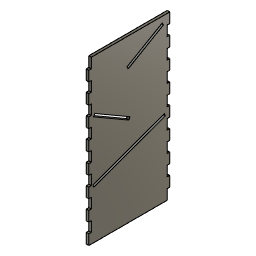
Dice Tower (Right Side) (Autodesk Fusion 360 design; units mm, degrees)
Autodesk Fusion 360 part; units mm, degrees
note: some values were not read from the file. Set by a fixed rule: which sketch regions a step uses.
sketch "Sketch1" plane through (0, 0, 0) normal (1, 0, 0) x (0, 1, 0)
  line L0 (98.425, 139.7) -> (101.6, 139.7)
  line L1 (0, 101.6) -> (0, 114.3)
  line L2 (0, 127) -> (0, 139.7)
  line L3 (98.425, 114.3) -> (101.6, 114.3)
  line L4 (0, 127) -> (3.175, 127)
  line L5 (101.6, 101.6) -> (101.6, 88.9)
  line L6 (0, 101.6) -> (3.175, 101.6)
  line L7 (98.425, 0) -> (98.425, 203.2)
  line L8 (98.425, 114.3) -> (98.425, 101.6)
  line L9 (98.425, 88.9) -> (101.6, 88.9)
  line L10 (101.6, 0) -> (100.0125, 0)
  line L11 (98.425, 127) -> (101.6, 127)
  line L12 (98.425, 101.6) -> (101.6, 101.6)
  line L13 (98.425, 95.25) -> (98.425, 88.9)
  line L14 (3.175, 0) -> (3.175, 203.2)
  line L15 (101.6, 127) -> (101.6, 114.3)
  line L16 (3.175, 127) -> (3.175, 114.3)
  line L17 (3.175, 88.9) -> (0, 88.9)
  line L18 (98.425, 139.7) -> (98.425, 127)
  line L19 (3.175, 114.3) -> (0, 114.3)
  line L20 (3.175, 12.7) -> (3.175, 0)
  line L21 (3.175, 190.5) -> (3.175, 177.8)
  line L22 (3.175, 177.8) -> (0, 177.8)
  line L23 (101.6, 50.8) -> (101.6, 38.1)
  line L24 (3.175, 50.8) -> (3.175, 38.1)
  line L25 (98.425, 152.4) -> (101.6, 152.4)
  line L26 (98.425, 50.8) -> (101.6, 50.8)
  line L27 (98.425, 152.4) -> (98.425, 139.7)
  line L28 (3.175, 139.7) -> (0, 139.7)
  line L29 (0, 139.7) -> (0, 127)
  line L30 (3.175, 101.6) -> (3.175, 88.9)
  line L31 (98.425, 101.6) -> (98.425, 95.25)
  line L32 (98.425, 203.2) -> (98.425, 190.5)
  line L33 (101.6, 152.4) -> (101.6, 139.7)
  line L34 (101.6, 203.2) -> (101.6, 190.5)
  line L35 (3.175, 203.2) -> (3.175, 190.5)
  line L36 (0, 0) -> (11.0998, 0)
  line L37 (98.425, 177.8) -> (98.425, 165.1)
  line L38 (98.425, 127) -> (98.425, 114.3)
  line L39 (0, 165.1) -> (0, 152.4)
  line L40 (11.0998, 0) -> (6.0198, 0)
  line L41 (98.425, 88.9) -> (98.425, 76.2)
  line L42 (0, 38.1) -> (3.175, 38.1)
  line L43 (98.425, 38.1) -> (98.425, 25.4)
  line L44 (101.6, 177.8) -> (101.6, 165.1)
  line L45 (98.425, 12.7) -> (101.6, 12.7)
  line L46 (0, 177.8) -> (0, 190.5)
  line L47 (98.425, 177.8) -> (101.6, 177.8)
  line L48 (0, 76.2) -> (0, 88.9)
  line L49 (0, 114.3) -> (0, 101.6)
  line L50 (3.175, 190.5) -> (0, 190.5)
  line L51 (98.425, 190.5) -> (101.6, 190.5)
  line L52 (101.6, 0) -> (0, 0)
  line L53 (98.425, 38.1) -> (101.6, 38.1)
  line L54 (90.5002, 0) -> (95.5802, 0)
  line L55 (3.175, 203.2) -> (101.6, 203.2)
  line L56 (98.425, 76.2) -> (101.6, 76.2)
  line L57 (98.425, 165.1) -> (101.6, 165.1)
  line L58 (98.425, 63.5) -> (98.425, 50.8)
  line L59 (98.425, 25.4) -> (101.6, 25.4)
  line L60 (0, 0) -> (0, 12.7)
  line L61 (3.175, 63.5) -> (0, 63.5)
  line L62 (98.425, 63.5) -> (101.6, 63.5)
  line L63 (0, 152.4) -> (0, 165.1)
  line L64 (0, 152.4) -> (3.175, 152.4)
  line L65 (0, 25.4) -> (0, 38.1)
  line L66 (0, 0) -> (12.065, 0)
  line L67 (3.175, 50.8) -> (0, 50.8)
  line L68 (101.6, 203.2) -> (98.425, 203.2)
  line L69 (98.425, 190.5) -> (98.425, 177.8)
  line L70 (101.6, 76.2) -> (101.6, 63.5)
  line L71 (101.6, 0) -> (90.5002, 0)
  line L72 (3.175, 25.4) -> (3.175, 12.7)
  line L73 (98.425, 25.4) -> (98.425, 12.7)
  line L74 (3.175, 38.1) -> (3.175, 25.4)
  line L75 (0, 12.7) -> (3.175, 12.7)
  line L76 (0, 50.8) -> (0, 63.5)
  line L77 (0, 25.4) -> (3.175, 25.4)
  line L78 (3.175, 177.8) -> (3.175, 165.1)
  line L79 (101.6, 0) -> (98.425, 0)
  line L80 (101.6, 0) -> (85.725, 0)
  line L81 (101.6, 25.4) -> (101.6, 12.7)
  line L82 (3.175, 76.2) -> (0, 76.2)
  line L83 (98.425, 165.1) -> (98.425, 152.4)
  line L84 (3.175, 63.5) -> (3.175, 50.8)
  line L85 (3.175, 152.4) -> (3.175, 139.7)
  line L86 (98.425, 76.2) -> (98.425, 63.5)
  line L87 (3.175, 165.1) -> (0, 165.1)
  line L88 (98.425, 50.8) -> (98.425, 38.1)
  line L89 (3.175, 76.2) -> (3.175, 63.5)
  line L90 (0, 0) -> (3.175, 0)
  line L91 (3.175, 88.9) -> (3.175, 76.2)
  line L92 (98.425, 203.2) -> (98.425, 177.8)
  line L93 (3.175, 0) -> (3.175, 59.055)
  line L94 (7.62, 139.7) -> (51.5837, 114.2474)
  line L95 (49.9801, 111.4777) -> (6.0165, 136.9303)
  line L96 (6.0165, 136.9303) -> (7.62, 139.7)
  line L97 (93.7411, 193.04) -> (49.7434, 167.6463)
  line L98 (92.1413, 195.8119) -> (93.7411, 193.04)
  line L99 (48.1436, 170.4182) -> (92.1413, 195.8119)
  line L100 (3.175, 60.2676) -> (4.1957, 60.2676)
  line L101 (4.1957, 60.2676) -> (6.35, 60.2676)
  line L102 (6.35, 60.2676) -> (95.8689, 92.8088)
  line L103 (94.7755, 95.8167) -> (5.2566, 63.2754)
  line L104 (49.9801, 111.4777) -> (50.2, 111.3504)
  line L105 (50.2, 111.3504) -> (51.8035, 114.1201)
  line L106 (51.8035, 114.1201) -> (51.5837, 114.2474)
  line L107 (95.8689, 92.8088) -> (96.1076, 92.8956)
  line L108 (96.1076, 92.8956) -> (95.0142, 95.9034)
  line L109 (95.0142, 95.9034) -> (94.7755, 95.8167)
  line L110 (49.7434, 167.6463) -> (49.5234, 167.5194)
  line L111 (49.5234, 167.5194) -> (47.9236, 170.2912)
  line L112 (47.9236, 170.2912) -> (48.1436, 170.4182)
  line L113 (5.2566, 63.2754) -> (6.35, 60.2676)
  dimension "d9" = 11.0998
  dimension "d10" = 11.0998
  dimension "d14" = 5.08
  dimension "d15" = 5.08
  dimension "d27" = 3.175
  dimension "d28" = 3.175
  dimension "d40" = 3.175
  dimension "d41" = 3.175
  dimension "d42" = 12.7
  dimension "d43" = 12.7
  dimension "d44" = 12.7
  dimension "d45" = 12.7
  dimension "d46" = 12.7
  dimension "d47" = 12.7
  dimension "d48" = 12.7
  dimension "d49" = 12.7
  dimension "d50" = 6.35
  dimension "d51" = 6.35
  dimension "d52" = 12.7
  dimension "d53" = 12.7
  dimension "d54" = 12.7
  dimension "d55" = 12.7
  dimension "d56" = 12.7
  dimension "d57" = 12.7
  dimension "d74" = 59.055
  dimension "d78" = 50.8
  dimension "d79" = 3.2004
  dimension "d80" = 50.8
  dimension "d81" = 50.8
  dimension "d82" = 3.2004
  dimension "d83" = 50.8
  dimension "d84" = 95.25
  dimension "d85" = 3.2004
  dimension "d86" = 95.25
  dimension "d87" = 0.254
  dimension "d88" = 0.254
  dimension "d89" = 3.2004
  dimension "d90" = 0.254
  dimension "d91" = 3.2004
  constraint coincident L36.start L52.end
  constraint vertical L60
  constraint perpendicular L55 L60
  constraint perpendicular L34 L55
  constraint perpendicular L52 L60
  constraint perpendicular L60 L66
  constraint perpendicular L34 L80
  constraint perpendicular L10 L34
  constraint coincident L54.start L52
  constraint perpendicular L36 L60
  constraint perpendicular L50 L60
  constraint perpendicular L21 L50
  constraint coincident L22.end L60
  constraint perpendicular L22 L60
  constraint perpendicular L22 L78
  constraint perpendicular L60 L87
  constraint collinear L46 L60
  constraint perpendicular L39 L87
  constraint perpendicular L39 L64
  constraint parallel L66 L90
  constraint perpendicular L14 L55
  constraint perpendicular L64 L85
  constraint perpendicular L28 L60
  constraint perpendicular L28 L29
  constraint coincident L4.end L14
  constraint perpendicular L4 L14
  constraint perpendicular L4 L16
  constraint perpendicular L16 L19
  constraint perpendicular L19 L49
  constraint midpoint L6.end L14
  constraint perpendicular L6 L14
  constraint perpendicular L6 L30
  constraint parallel L14 L91
  constraint parallel L14 L89
  constraint parallel L14 L84
  constraint parallel L14 L24
  constraint parallel L24 L74
  constraint parallel L14 L72
  constraint perpendicular L17 L60
  constraint coincident L48.start L60
  constraint perpendicular L60 L82
  constraint perpendicular L60 L61
  constraint coincident L67.end L60
  constraint perpendicular L60 L67
  constraint coincident L65.start L60
  constraint collinear L60 L63
  constraint collinear L2 L60
  constraint collinear L1 L60
  constraint collinear L48 L60
  constraint collinear L60 L76
  constraint collinear L60 L65
  constraint perpendicular L34 L68
  constraint perpendicular L34 L79
  constraint perpendicular L32 L55
  constraint perpendicular L34 L51
  constraint perpendicular L51 L69
  constraint coincident L44.start L34
  constraint perpendicular L34 L47
  constraint perpendicular L37 L47
  constraint coincident L44.end L34
  constraint perpendicular L34 L57
  constraint perpendicular L57 L83
  constraint coincident L25.end L34
  constraint perpendicular L25 L34
  constraint perpendicular L25 L27
  constraint coincident L0.end L34
  constraint perpendicular L0 L34
  constraint perpendicular L0 L18
  constraint coincident L11.end L34
  constraint perpendicular L11 L34
  constraint perpendicular L11 L38
  constraint coincident L3.end L34
  constraint perpendicular L3 L34
  constraint perpendicular L3 L8
  constraint perpendicular L12 L34
  constraint perpendicular L12 L31
  constraint parallel L7 L13
  constraint coincident L5.end L34
  constraint perpendicular L9 L34
  constraint perpendicular L9 L41
  constraint coincident L56.end L34
  constraint perpendicular L34 L56
  constraint perpendicular L56 L86
  constraint coincident L62.end L34
  constraint perpendicular L34 L62
  constraint perpendicular L58 L62
  constraint coincident L23.start L34
  constraint perpendicular L26 L34
  constraint perpendicular L26 L88
  constraint coincident L23.end L34
  constraint perpendicular L34 L53
  constraint perpendicular L43 L53
  constraint perpendicular L43 L59
  constraint perpendicular L59 L73
  constraint perpendicular L45 L73
  constraint collinear L34 L44
  constraint coincident L5.start L34
  constraint collinear L33 L44
  constraint collinear L15 L33
  constraint collinear L5 L15
  constraint collinear L5 L70
  constraint collinear L23 L70
  constraint collinear L23 L81
  constraint coincident L84 L93.end
  constraint coincident L84 L100.start
  constraint perpendicular L84 L100
  constraint perpendicular L93 L101
  constraint perpendicular L95 L105
  constraint parallel L102 L107
  constraint perpendicular L107 L108
  constraint parallel L97 L110
  constraint perpendicular L110 L111
  constraint perpendicular L111 L112
  constraint perpendicular L102 L113
  measures "d9" distance of L10.start L54.start
  measures "d10" distance of L36.start L36.end
  measures "d14" distance of L36.end L40.end
  measures "d15" distance of L54.end L54.start
  measures "d27" distance of L39.end L64.end
  measures "d28" distance of L36.start L14.start
  measures "d40" distance of L7.end L34.start
  measures "d41" distance of L7.start L10.start
  measures "d42" distance of L7.end L32.end
  measures "d43" distance of L32.end L37.start
  measures "d44" distance of L37.end L37.start
  measures "d45" distance of L25.start L37.end
  measures "d46" distance of L0.start L25.start
  measures "d47" distance of L0.start L11.start
  measures "d48" distance of L3.start L11.start
  measures "d49" distance of L8.end L3.start
  measures "d50" distance of L8.end L13.start
  measures "d51" distance of L13.start L9.start
  measures "d52" distance of L9.start L41.end
  measures "d53" distance of L41.end L58.start
  measures "d54" distance of L58.start L26.start
  measures "d55" distance of L26.start L43.start
  measures "d56" distance of L43.end L43.start
  measures "d57" distance of L43.end L45.start
  measures "d74" distance of L14.start L93.end
  measures "d78" distance of L94.start L94.end
  measures "d79" distance of L95.start L94.end
  measures "d80" distance of L95.start L95.end
  measures "d81" distance of L97.start L97.end
  measures "d82" distance of L99.start L97.end
  measures "d83" distance of L98.start L99.start
  measures "d84" distance of L101.end L102.end
  measures "d85" distance of L102.end L103.start
  measures "d86" distance of L103.start L103.end
  measures "d87" distance of L95.start L104.end
  measures "d88" distance of L102.end L107.end
  measures "d89" distance of L107.end L108.end
  measures "d90" distance of L97.end L110.end
  measures "d91" distance of L110.end L111.end
extrude "Extrude1" add sketch "Sketch1" along normal blind 3.175
sketch "Sketch2" plane through (0, 0, 0) normal (1, 0, 0) x (0, 1, 0)
equation "d9 = 0.5 in - 0.063 in"
